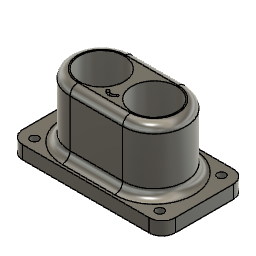
GoggleOccluder (Autodesk Fusion 360 design; units mm, degrees)
Autodesk Fusion 360 part; units mm, degrees
sketch "Sketch1" plane through (0, 0, 0) normal (0, 1, 0) x (1, 0, 0)
  line L0 (29, 16) -> (-29, 16)
  line L1 (-29, 16) -> (-29, -16)
  line L2 (-29, -16) -> (29, -16)
  line L3 (29, -16) -> (29, 16)
  line L4 (23.8029, 11.7183) -> (-23.8029, 11.7183) construction
  line L5 (-23.8029, 11.7183) -> (-23.8029, -11.7183) construction
  line L6 (-23.8029, -11.7183) -> (23.8029, -11.7183) construction
  line L7 (23.8029, -11.7183) -> (23.8029, 11.7183) construction
  line L8 (23.8029, 11.7183) -> (-23.8029, -11.7183) construction
  line L9 (-23.8029, 11.7183) -> (23.8029, -11.7183) construction
  circle A0 centre (-23.8029, 11.7183) radius 1.55
  circle A1 centre (23.8029, 11.7183) radius 1.55
  circle A2 centre (23.8029, -11.7183) radius 1.55
  circle A3 centre (-23.8029, -11.7183) radius 1.55
  line L10 (-10, 0) -> (10, 0) construction
  circle A4 centre (-10, 0) radius 8.5
  circle A5 centre (10, 0) radius 8.5
  line L11 (0, 11.7183) -> (0, 16) construction
  dimension "d2" = 32
  dimension "d4" = 3.1
  dimension "d5" = 17
  dimension "d6" = 20
  dimension "d7" = 58
  constraint horizontal L0
  constraint perpendicular L0 L1
  constraint parallel L0 L2
  constraint parallel L1 L3
  constraint horizontal L4
  constraint perpendicular L4 L5
  constraint parallel L4 L6
  constraint parallel L5 L7
  constraint coincident L8 origin
  constraint coincident L9 origin
  constraint coincident L4.end L5.start
  constraint coincident L4.start L7.end
  constraint coincident L6.end L7.start
  constraint coincident L5.end L6.start
  constraint equal A0 A1
  constraint equal A1 A2
  constraint equal A2 A3
  constraint horizontal L10
  constraint midpoint origin L10
  constraint coincident L10.start A4.centre
  constraint coincident L10.end A5.centre
  constraint equal A4 A5
  constraint midpoint L4 L11.start
  constraint coincident L0 L11.end
  constraint perpendicular L0 L11
  constraint midpoint L0 L11.end
  measures "d2" distance of L0.end L1.end
  measures "d4" diameter of A0
  measures "d5" diameter of A4
  measures "d6" distance of L10.start L10.end
  measures "d7" distance of L1 L3
extrude "Extrude1" add sketch "Sketch1" along normal blind 5
sketch "Sketch2" plane through (0, 5, 0) normal (0, 1, 0) x (-1, 0, 0)
  circle A0 centre (-23.8029, -11.7183) radius 1.55
  circle A1 centre (23.8029, -11.7183) radius 1.55
  circle A2 centre (-23.8029, 11.7183) radius 1.55
  circle A3 centre (23.8029, 11.7183) radius 1.55
  circle A4 centre (10, 0) radius 8.5
  circle A5 centre (-10, 0) radius 8.5
  line L0 (-29, 16) -> (-29, -16)
  line L1 (-29, -16) -> (29, -16)
  line L2 (29, -16) -> (29, 16)
  line L3 (29, 16) -> (-29, 16)
  line L4 (10, 12) -> (-10, 12)
  arc A6 (-10, 12) -> (-10, -12) centre (-10, 0) ccw
  line L5 (-10, -12) -> (10, -12)
  arc A7 (10, -12) -> (10, 12) centre (10, 0) ccw
  line L6 (10, 0) -> (-10, 0) construction
  dimension "d10" = 20
  dimension "d11" = 12
  constraint tangent L4 A6
  constraint tangent A6 L5
  constraint parallel L4 L5
  constraint tangent L5 A7
  constraint tangent L4 A7
  constraint horizontal L6
  constraint midpoint L6 origin
  measures "d10" distance of A4.centre A5.centre
  measures "d11" radius of A6
extrude "Extrude2" add sketch "Sketch2" along normal blind 24 contours L4 A6 L5 A7
fillet "Fillet1" radius 5 4 edges at (-29, 2.5, 16) (-29, 2.5, -16) (29, 2.5, -16) (29, 2.5, 16)
fillet "Fillet2" radius 3 4 faces at (-3.3333, 13, 12) (20.0803, 13, -6.5106) (3.3333, 13, -12) (-17.2457, 21, -9.5656)
sketch "Sketch3" plane through (0, 29, 0) normal (0, 1, 0) x (-1, 0, 0)
  circle A0 centre (-10, 0) radius 8.5
  circle A1 centre (10, 0) radius 8.5
  line L0 (10, 9) -> (-10, 9)
  arc A2 (-10, 9) -> (-10, -9) centre (-10, 0) ccw
  line L1 (-10, -9) -> (10, -9)
  arc A3 (10, -9) -> (10, 9) centre (10, 0) ccw
  arc A4 (1.2397, 5.6527) -> (-1.2397, 5.6527) centre (0, 5) ccw
  arc A5 (1.2397, 5.6527) -> (2.1245, 6.1185) centre (1.6821, 5.8856) ccw
  arc A6 (2.1245, 6.1185) -> (-2.1245, 6.1185) centre (0, 5) ccw
  arc A7 (-2.1245, 6.1185) -> (-1.2397, 5.6527) centre (-1.6821, 5.8856) ccw
  arc A8 (1.6821, 5.8856) -> (-1.6821, 5.8856) centre (0, 5) ccw construction
  line L2 (0, 5) -> (0, 0) construction
  line L3 (1.6821, 5.8856) -> (-1.6821, 5.8856) construction
  dimension "d18" = 0.5
  dimension "d19" = 5
  constraint tangent A4 A5
  constraint tangent A5 A6
  constraint tangent A6 A7
  constraint tangent A4 A7
  constraint coincident A4.centre A6.centre
  constraint coincident L2.end origin
  constraint vertical L2
  constraint coincident A5.centre A8.start
  constraint coincident A7.centre A8.end
  constraint horizontal L3
  measures "d18" radius of A7
  measures "d19" distance of A4.centre L2.end
extrude "Extrude3" cut sketch "Sketch3" against normal blind 1 contours A4 A5 A6 A7
